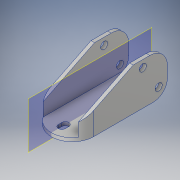
# Autodesk Inventor part: CAR_048_NewCarouselTensioner1.5UChannel
Saved by Autodesk Inventor 2018 (Build 220112000, 112)
## iProperties
Created: 2020-02-15
Part Number: CAR_048_NewCarouselTensioner1.5UChannel
Material: Aluminum 6061
Document SubType Name: Modeling
Designer: user
Density: 2.7 g/cm^3
Appearance: Aluminum - Flat
Mass: 94.0208 g
Surface Area: 232.661 cm^2
Volume: 34.8225 cm^3
Author: user
Autodesk Inventor part; units mm, degrees
ref_plane "YZ Plane" through (0, 0, 0) normal (1, 0, 0) x (0, 1, 0)
ref_plane "XZ Plane" through (0, 0, 0) normal (0, 1, 0) x (-1, 0, 0)
ref_plane "XY Plane" through (0, 0, 0) normal (0, 0, 1) x (1, 0, 0)
sketch "Sketch1" plane through (0, 0, 0) normal (0, 0, 1) x (1, 0, 0)
  line L0 (0, 0) -> (3.175, 0)
  line L1 (3.175, 0) -> (3.175, 38.1)
  line L2 (3.175, 38.1) -> (0, 38.1)
  line L3 (0, 38.1) -> (0, 0)
  line L4 (0, 0) -> (38.1, 0)
  line L5 (38.1, 0) -> (38.1, 3.175)
  line L6 (38.1, 3.175) -> (0, 3.175)
  line L7 (0, 3.175) -> (0, 0)
  line L8 (38.1, 0) -> (34.925, 0)
  line L9 (34.925, 0) -> (34.925, 38.1)
  line L10 (34.925, 38.1) -> (38.1, 38.1)
  line L11 (38.1, 38.1) -> (38.1, 0)
  dimension "d0" = 3.175
  dimension "d1" = 38.1
  dimension "d2" = 38.1
  dimension "d3" = 3.175
  dimension "d4" = 3.175
  dimension "d5" = 38.1
  constraints: 24 end point, 6 parallel, 3 horizontal, 3 perpendicular
  measures "d0" distance of L2.end L1.end
  measures "d1" distance of L1.end L0.end
  measures "d2" distance of L6.end L5.end
  measures "d3" distance of L5.end L4.end
  measures "d4" distance of L9.end L10.end
  measures "d5" distance of L8.end L9.end
extrude "Extrusion1" add sketch "Sketch1" along normal blind 101.6
sketch "Sketch2" plane through (38.1, 0, 0) normal (1, 0, 0) x (0, 0, -1)
  line L0 (-101.6, 3.175) -> (0, 3.175) projected
  line L1 (0, 0) -> (0, 38.1) projected
  point P0 (-7.9375, 9.525)
  dimension "d8" = 6.35
  dimension "d9" = 7.9375
  measures "d8" distance from line of L0 point (-7.937, 9.525)
  measures "d9" distance from line of point (-7.937, 9.525) L1
hole "Hole1" at (38.1, 9.525, 7.9375) direction (-1, 0, 0) diameter 6.35 end through all
sketch "Sketch3" plane through (38.1, 0, 0) normal (1, 0, 0) x (0, 0, -1)
  line L0 (0, 38.1) -> (-101.6, 38.1) projected
  line L1 (0, 0) -> (0, 38.1) projected
  point P0 (-22.225, 31.75)
  dimension "d17" = 6.35
  dimension "d18" = 22.225
  measures "d17" distance from line of L0 point (-22.225, 31.75)
  measures "d18" distance from line of point (-22.225, 31.75) L1
hole "Hole2" at (38.1, 31.75, 22.225) direction (-1, 0, 0) diameter 6.35 end through all
ref_plane "Work Plane1" through (19.05, 3.175, 0) normal (-1, 0, 0) x (0, 0, 1)
fillet "Fillet1" radius 12.7 1 edges at (19.05, 0, 0)
sketch "Sketch4" plane through (0, 0, 101.6) normal (-1, 0, 0) x (0, 0, 1)
  line L0 (-78.4449, 41.9138) -> (31.1063, -12.1864)
  line L1 (31.1063, -12.1864) -> (58.2522, 42.7832)
  line L2 (58.2522, 42.7832) -> (-51.299, 96.8833)
  line L3 (-51.299, 96.8833) -> (-78.4449, 41.9138)
  arc A0 (-101.6, 12.7) -> (-88.9, 0) centre (-88.9, 12.7) ccw projected
  line L4 (-88.9, 0) -> (0, 0) projected
  line L5 (0, 38.1) -> (0, 0) projected
  line L6 (-101.6, 38.1) -> (0, 38.1) projected
  line L7 (-101.6, 38.1) -> (-101.6, 12.7) projected
  circle A1 centre (-79.375, 31.75) radius 3.175 projected
  circle A2 centre (-93.6625, 9.525) radius 3.175 projected
  line L8 (-97.3003, 3.175) -> (0, 3.175) projected
  point P0 (-101.6, 0)
  dimension "d27" = 9.525
  dimension "d28" = 6.35
  constraints: 8 end point, 2 parallel, 1 perpendicular, 1 point on line
  measures "d27" distance from line of A1.centre L0
  measures "d28" diameter of A1
extrude "Extrusion2" cut sketch "Sketch4" against normal through all contours L5 L6 L0 L3 L2 L1 | L0 L6 L5
fillet "Fillet2" radius 15.875 2 edges at (1.5875, 38.1, 0) (36.5125, 38.1, 0)
sketch "Sketch5" plane through (0, 0, 101.6) normal (0, -1, 0) x (1, 0, 0)
  line L0 (0, -88.9) -> (0, 0) projected
  point P0 (0, -101.6)
  point P1 (19.05, -25.4)
  dimension "d32" = 19.05
  dimension "d40" = 76.2
  measures "d32" distance from line of point (19.05, -25.4) L0
  measures "d40" vertical distance of point (0, -101.6) point (19.05, -25.4)
hole "Hole3" at (19.05, 0, 76.2) direction (0, 1, 0) diameter 6.35 end through all
sketch "Sketch6" plane through (0, 0, 101.6) normal (0, -1, 0) x (1, 0, 0)
  circle A0 centre (19.05, -25.4) radius 3.175
  circle A1 centre (19.05, -25.4) radius 3.175 projected
  line L0 (38.1, -88.9) -> (0, -88.9) projected
  line L1 (38.1, -88.9) -> (38.1, 0) projected
  line L2 (0, 0) -> (38.1, 0) projected
  line L3 (0, -88.9) -> (0, 0) projected
  line L4 (-11.1164, -15.875) -> (47.1756, -15.875)
  line L5 (47.1756, -15.875) -> (47.1756, 8.1032)
  line L6 (47.1756, 8.1032) -> (-11.1164, 8.1032)
  line L7 (-11.1164, 8.1032) -> (-11.1164, -15.875)
  point P0 (0, -101.6)
  dimension "d41" = 9.525
  dimension "d42" = 6.35
  constraints: 8 end point, 2 parallel, 1 centre point, 1 concentric, 1 horizontal, 1 perpendicular
  measures "d41" distance from line of L4 A0.centre
  measures "d42" diameter of A0
extrude "Extrusion3" cut sketch "Sketch6" against normal through all contours L4 L3 L2 L1 | L1 L2 L3 L4 L7 L6 L5
fillet "Fillet3" radius 19.05 2 edges at (0, 5.5073, 85.725) (38.1, 5.5073, 85.725)
sketch "Sketch7" plane through (0, 0, 12.7) normal (0, -1, 0) x (1, 0, 0)
  circle A0 centre (19.05, 63.5) radius 3.175 projected
  line L0 (19.05, 63.5) -> (19.05, 60.325) construction
  line L1 (15.875, 63.5) -> (15.875, 60.325)
  line L2 (22.225, 60.325) -> (22.225, 63.5)
  arc A1 (22.225, 63.5) -> (15.875, 63.5) centre (19.05, 63.5) ccw
  arc A2 (15.875, 60.325) -> (22.225, 60.325) centre (19.05, 60.325) ccw
  point P0 (0, -12.7)
  point P1 (19.05, 61.9125)
  dimension "d46" = 3.175
  constraints: 8 end point, 4 point on circle, 4 tangent, 2 centre point, 1 concentric, 1 midpoint, 1 parallel, 1 vertical
  measures "d46" distance of L1.start L1.end
extrude "Extrusion4" cut sketch "Sketch7" against normal blind 25.4 contours L2 A2 L1 A0
body "Solid1"
